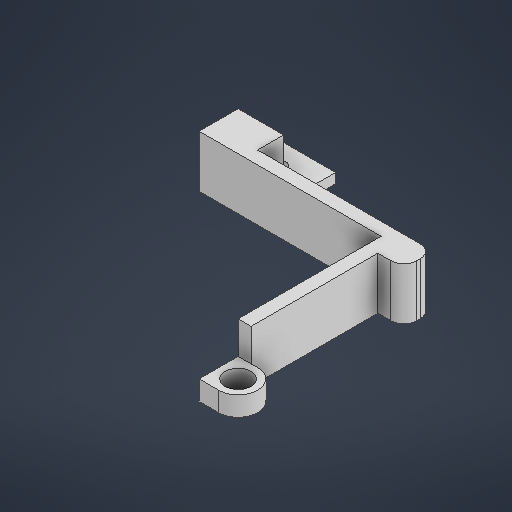
# Autodesk Inventor part: prawascianakolo
Saved by Autodesk Inventor 2026.2 (Build 302298010, 298A)
## iProperties
Created: 2026-04-27
Part Number: prawascianakolo
Material: Ogólny
Document SubType Name: Modeling
Designer: karol
Density: 1 g/cm^3
Appearance: Domyślna
Author: karol
Autodesk Inventor part; units mm, degrees
ref_plane "YZ Plane" through (0, 0, 0) normal (1, 0, 0) x (0, 1, 0)
ref_plane "XZ Plane" through (0, 0, 0) normal (0, 1, 0) x (-1, 0, 0)
ref_plane "XY Plane" through (0, 0, 0) normal (0, 0, 1) x (1, 0, 0)
sketch "Szkic1" plane through (0, 0, 0) normal (0, 1, 0) x (-1, 0, 0)
  line L0 (0, 0) -> (3, 0)
  line L1 (3, 0) -> (3, -25)
  line L2 (3, -25) -> (0, -25)
  line L3 (0, -25) -> (0, 0)
  line L4 (3, -25) -> (31, -25)
  line L5 (31, -25) -> (31, -22)
  line L6 (31, -22) -> (3, -22)
  line L7 (3, -22) -> (3, -25)
  point P0 (3, -22)
  dimension "d0" = 3
  dimension "d1" = 25
  dimension "d2" = 28
  dimension "d3" = 3
  constraints: 16 end point, 4 parallel, 2 horizontal, 2 perpendicular
  measures "d0" distance of L1.end L2.end
  measures "d1" distance of L0.end L1.end
  measures "d2" distance of L6.end L5.end
  measures "d3" distance of L5.end L4.end
extrude "Wyciągnięcie proste1" add sketch "Szkic1" along normal blind 8
sketch "Szkic2" plane through (0, 0, 0) normal (1, 0, 0) x (0, 0, -1)
  line L0 (0, 0) -> (0, 8) projected
  line L1 (0, 8) -> (5, 8)
  line L2 (5, 8) -> (5, 0)
  line L3 (5, 0) -> (0, 0)
  line L4 (0, 0) -> (0, 8)
  dimension "d6" = 5
  dimension "d7" = 8
  constraints: 8 end point, 2 parallel, 1 horizontal, 1 perpendicular
  measures "d6" distance of L2.end L3.end
  measures "d7" distance of L1.end L2.end
extrude "Wyciągnięcie proste2" add sketch "Szkic2" along normal blind 3
sketch "Szkic6" plane through (0, 8, 0) normal (0, 1, 0) x (1, 0, 0)
  line L0 (-31, 22) -> (-3, 22) projected
  line L1 (0, 25) -> (-31, 25) projected
  line L2 (-3, 22) -> (0, 22)
  line L3 (0, 22) -> (0, 25)
  line L4 (0, 25) -> (-3, 25)
  line L5 (-3, 25) -> (-3, 22)
  line L6 (-3, 25) -> (3, 25)
  line L7 (3, 25) -> (3, 19)
  line L8 (3, 19) -> (-3, 19)
  line L9 (-3, 19) -> (-3, 25)
  point P0 (0, 0)
  dimension "d19" = 6
  dimension "d20" = 6
  constraints: 16 end point, 4 parallel, 2 horizontal, 2 perpendicular
  measures "d19" distance of L7.end L8.end
  measures "d20" distance of L6.end L7.end
extrude "Wyciągnięcie proste6" add sketch "Szkic6" against normal blind 8 contours L6 L7 L8 L9 L2 L3
sketch "Szkic7" plane through (0, 8, 0) normal (0, 1, 0) x (1, 0, 0)
  line L0 (3, 19) -> (3, 25) projected
  line L1 (-31, 25) -> (3, 25) projected
  line L2 (-3, 22) -> (-3, 0) projected
  circle A0 centre (0, 22) radius 1.5
  point P0 (0, 0)
  dimension "d23" = 3
  dimension "d42" = 3
  dimension "d43" = 3
  constraints: 1 centre point
  measures "d23" diameter of A0
  measures "d42" distance from line of L1 A0.centre
  measures "d43" distance from line of L2 A0.centre
extrude "Wyciągnięcie proste7" cut sketch "Szkic7" against normal blind 8
sketch "Szkic8" plane through (0, 8, 0) normal (0, 1, 0) x (1, 0, 0)
  circle A0 centre (0, 22) radius 1.5 projected
  circle A1 centre (0, 22) radius 2
  point P0 (0, 0)
  constraints: 1 centre point, 1 coincident
extrude "Wyciągnięcie proste8" add sketch "Szkic8" against normal blind 3 contours A0
sketch "Szkic9" plane through (0, 8, 0) normal (0, 1, 0) x (1, 0, 0)
  line L0 (-31, 25) -> (-31, 22) projected
  line L1 (3, 19) -> (3, 25) projected
  line L2 (-31, 25) -> (3, 25)
  line L3 (3, 25) -> (3, 24)
  line L4 (3, 24) -> (-31, 24)
  line L5 (-31, 24) -> (-31, 25)
  point P0 (0, 0)
  dimension "d28" = 1
  constraints: 8 end point, 2 parallel, 1 horizontal, 1 perpendicular, 1 point on line
  measures "d28" distance of L2.end L3.end
extrude "Wyciągnięcie proste9" cut sketch "Szkic9" against normal blind 8
sketch "Szkic10" plane through (0, 0, -5) normal (0, 0, -1) x (-1, 0, 0)
  line L0 (0, 0) -> (0, 8) projected
  line L1 (-3, 8) -> (-3, 0) projected
  line L2 (0, 0) -> (-3, 0)
  line L3 (-3, 0) -> (-3, 8)
  line L4 (-3, 8) -> (0, 8)
  line L5 (0, 8) -> (0, 0)
  point P0 (-3, 0)
  constraints: 8 end point, 2 parallel, 1 horizontal, 1 perpendicular
extrude "Wyciągnięcie proste10" cut sketch "Szkic10" against normal blind 3.7
sketch "Szkic11" plane through (0, 8, -19) normal (0, 0, 1) x (1, 0, 0)
  line L0 (-3, 0) -> (3, 0) projected
  line L1 (3, -8) -> (0, -8) projected
  line L2 (0, 0) -> (3, 0)
  line L3 (3, 0) -> (3, -8)
  line L4 (3, -8) -> (0, -8)
  line L5 (0, -8) -> (0, 0)
  constraints: 8 end point, 2 parallel, 1 horizontal, 1 midpoint, 1 perpendicular
extrude "Wyciągnięcie proste11" cut sketch "Szkic11" against normal blind 0.5
sketch "Szkic12" plane through (3, 8, -24) normal (0, 0, -1) x (-1, 0, 0)
  line L0 (0, -8) -> (0, 0) projected
  line L1 (6, 0) -> (0, 0) projected
  line L2 (0, -8) -> (6, -8)
  line L3 (6, -8) -> (6, 0)
  line L4 (6, 0) -> (0, 0)
  line L5 (0, 0) -> (0, -8)
  point P0 (3, -8)
  constraints: 8 end point, 2 parallel, 1 horizontal, 1 perpendicular
extrude "Wyciągnięcie proste12" add sketch "Szkic12" along normal blind 0.5
sketch "Szkic13" plane through (0, 0, -1.3) normal (1, 0, 0) x (0, 0, -1)
  line L0 (0, 0) -> (18.2, 0) projected
  line L1 (0, 8) -> (18.2, 8) projected
  line L2 (0, 0) -> (18.2, 0)
  line L3 (18.2, 0) -> (18.2, 8)
  line L4 (18.2, 8) -> (0, 8)
  line L5 (0, 8) -> (0, 0)
  point P0 (-1.3, 0)
  point P1 (18.2, 0)
  constraints: 8 end point, 2 parallel, 1 horizontal, 1 perpendicular
extrude "Wyciągnięcie proste13" cut sketch "Szkic13" against normal blind 1
sketch "Szkic14" plane through (3, 8, -24.5) normal (0, 0, -1) x (-1, 0, 0)
  line L0 (4, 0) -> (0, 0) projected
  line L1 (6, -8) -> (6, 0) projected
  line L2 (0, 0) -> (6, 0)
  line L3 (6, 0) -> (6, -8)
  line L4 (6, -8) -> (0, -8)
  line L5 (0, -8) -> (0, 0)
  point P0 (3, -8)
  constraints: 8 end point, 2 parallel, 1 horizontal, 1 perpendicular
extrude "Wyciągnięcie proste14" cut sketch "Szkic14" against normal blind 0.5
sketch "Szkic15" plane through (-3, 0, 0) normal (0, 0, 1) x (1, 0, 0)
  line L0 (6, 8) -> (6, 0) projected
  line L1 (0, 0) -> (0, 8) projected
  line L2 (6, 8) -> (0, 8)
  line L3 (0, 8) -> (0, 0)
  line L4 (0, 0) -> (6, 0)
  line L5 (6, 0) -> (6, 8)
  point P0 (3, 0)
  constraints: 8 end point, 2 parallel, 1 horizontal, 1 perpendicular
extrude "Wyciągnięcie proste15" add sketch "Szkic15" along normal blind 4.7
sketch "Szkic16" plane through (3, 0, 0) normal (1, 0, 0) x (0, 0, -1)
  line L0 (-4.7, 8) -> (-4.7, 0) projected
  line L1 (1.3, 0) -> (1.3, 8) projected
  line L2 (-4.7, 0) -> (1.3, 0)
  line L3 (1.3, 0) -> (1.3, 8)
  line L4 (1.3, 8) -> (-4.7, 8)
  line L5 (-4.7, 8) -> (-4.7, 0)
  point P0 (0, 0)
  constraints: 8 end point, 2 parallel, 1 horizontal, 1 perpendicular
extrude "Wyciągnięcie proste16" cut sketch "Szkic16" against normal blind 4
sketch "Szkic17" plane through (0, 8, 0) normal (0, 1, 0) x (1, 0, 0)
  line L0 (-1, 19.5) -> (-1, -4.7) projected
  line L1 (-3, -4.7) -> (-1, -4.7)
  line L2 (-1, -4.7) -> (-1, 0)
  line L3 (-1, 0) -> (-3, 0)
  line L4 (-3, 0) -> (-3, -4.7)
  line L5 (-3, 0) -> (3, 0)
  line L6 (3, 0) -> (3, -6)
  line L7 (3, -6) -> (-3, -6)
  line L8 (-3, -6) -> (-3, 0)
  point P0 (0, 0)
  dimension "d48" = 6
  dimension "d49" = 6
  constraints: 16 end point, 4 parallel, 2 horizontal, 2 perpendicular, 1 point on line
  measures "d48" distance of L6.end L7.end
  measures "d49" distance of L5.end L6.end
extrude "Wyciągnięcie proste17" cut sketch "Szkic17" against normal blind 5
sketch "Szkic18" plane through (0, 3, 0) normal (0, 1, 0) x (1, 0, 0)
  line L0 (-3, 0) -> (-1, 0) projected
  line L1 (-3, 0) -> (3, 0)
  line L2 (3, 0) -> (3, -6)
  line L3 (3, -6) -> (-3, -6)
  line L4 (-3, -6) -> (-3, 0)
  point P0 (0, 0)
  dimension "d52" = 6
  dimension "d53" = 6
  constraints: 8 end point, 2 parallel, 1 horizontal, 1 perpendicular
  measures "d52" distance of L2.end L3.end
  measures "d53" distance of L1.end L2.end
extrude "Wyciągnięcie proste18" add sketch "Szkic18" against normal blind 3
sketch "Szkic19" plane through (0, 3, 0) normal (0, 1, 0) x (1, 0, 0)
  circle A0 centre (0, -3) radius 2
  line L0 (-3, -6) -> (-3, 0) projected
  line L1 (-3, -6) -> (3, -6) projected
  point P0 (0, 0)
  dimension "d56" = 4
  dimension "d57" = 3
  dimension "d58" = 3
  constraints: 1 centre point
  measures "d56" diameter of A0
  measures "d57" distance from line of L0 A0.centre
  measures "d58" distance from line of L1 A0.centre
extrude "Wyciągnięcie proste19" cut sketch "Szkic19" against normal blind 3
sketch "Szkic20" plane through (-31, 0, -22) normal (0, 0, 1) x (1, 0, 0)
  line L0 (34, 8) -> (0, 8) projected
  line L1 (0, 8) -> (7, 8)
  line L2 (7, 8) -> (7, 4)
  line L3 (7, 4) -> (0, 4)
  line L4 (0, 4) -> (0, 8)
  point P0 (31, 0)
  point P1 (7, 8)
  dimension "d61" = 7
  dimension "d62" = 4
  constraints: 8 end point, 2 parallel, 1 horizontal, 1 perpendicular
  measures "d61" distance of L2.end L3.end
  measures "d62" distance of L1.end L2.end
extrude "Wyciągnięcie proste20" add sketch "Szkic20" along normal blind 4
sketch "Szkic21" plane through (-31, 0, -24) normal (-1, 0, 0) x (0, 0, 1)
  circle A0 centre (4, 6) radius 1.5
  line L0 (6, 8) -> (6, 4) projected
  line L1 (2, 4) -> (6, 4) projected
  point P0 (24, 0)
  point P1 (4, 4)
  dimension "d65" = 3
  dimension "d66" = 2
  dimension "d67" = 2
  constraints: 1 centre point, 1 midpoint
  measures "d65" diameter of A0
  measures "d66" distance from line of L0 A0.centre
  measures "d67" distance of point (4, 4) A0.centre
extrude "Wyciągnięcie proste21" cut sketch "Szkic21" against normal blind 6
sketch "Szkic22" plane through (3, 8, -24) normal (0, 0, -1) x (-1, 0, 0)
  line L0 (34, 0) -> (34, -8) projected
  line L1 (34, 0) -> (27, 0)
  line L2 (27, 0) -> (27, -4)
  line L3 (27, -4) -> (34, -4)
  line L4 (34, -4) -> (34, 0)
  point P0 (3, -8)
  dimension "d70" = 7
  dimension "d71" = 4
  constraints: 8 end point, 2 parallel, 1 horizontal, 1 perpendicular
  measures "d70" distance of L3.end L2.end
  measures "d71" distance of L2.end L1.end
extrude "Wyciągnięcie proste22" add sketch "Szkic22" along normal blind 4
sketch "Szkic23" plane through (-31, 0, -24) normal (-1, 0, 0) x (0, 0, 1)
  circle A0 centre (-2, 6) radius 1.5
  line L0 (-4, 8) -> (6, 8) projected
  line L1 (-4, 4) -> (-4, 8) projected
  line L2 (2, 0) -> (2, 8) projected
  line L3 (6, 8) -> (2, 8)
  line L4 (2, 8) -> (2, 4)
  line L5 (2, 4) -> (6, 4)
  line L6 (6, 4) -> (6, 8)
  point P0 (24, 0)
  point P1 (-4, 6)
  dimension "d74" = 3
  dimension "d75" = 2
  dimension "d76" = 2
  constraints: 8 end point, 2 midpoint, 2 parallel, 1 centre point, 1 horizontal, 1 perpendicular
  measures "d74" diameter of A0
  measures "d75" distance from line of L0 A0.centre
  measures "d76" distance of point (-4, 6) A0.centre
extrude "Wyciągnięcie proste23" cut sketch "Szkic23" against normal blind 7 contours L0 L6 L5 L2
extrude "Wyciągnięcie proste24" cut sketch "Szkic23" against normal blind 6 contours A0
sketch "Sketch24" plane through (3, 0, -24) normal (0, 0, -1) x (-1, 0, 0)
  line L0 (34, 4) -> (27, 4) projected
  line L1 (27, 4) -> (27, 8) projected
  line L2 (0, 8) -> (27, 8) projected
  line L3 (0, 0) -> (0, 8) projected
  line L4 (34, 0) -> (0, 0) projected
  line L5 (34, 4) -> (34, 0) projected
  point P0 (3, 0)
extrude "Extrusion25" add sketch "Sketch24" along normal blind 0.5
sketch "Szkic25" plane through (3, 0, -24.5) normal (0, 0, -1) x (-1, 0, 0)
  line L0 (27, 4) -> (34, 4) projected
  line L1 (27, 8) -> (27, 4) projected
  line L2 (27, 8) -> (0, 8) projected
  line L3 (0, 8) -> (0, 0) projected
  line L4 (0, 0) -> (34, 0) projected
  line L5 (34, 0) -> (34, 4) projected
  point P0 (3, 0)
extrude "Wyciągnięcie proste26" cut sketch "Szkic25" against normal blind 0.5
sketch "Szkic26" plane through (3, 0, -24) normal (0, 0, -1) x (-1, 0, 0)
  line L0 (34, 0) -> (6, 0) projected
  line L1 (34, 0) -> (24.5, 0)
  line L2 (24.5, 0) -> (24.5, 1.5)
  line L3 (24.5, 1.5) -> (34, 1.5)
  line L4 (34, 1.5) -> (34, 0)
  point P0 (3, 0)
  dimension "d85" = 9.5
  dimension "d86" = 1.5
  constraints: 8 end point, 2 parallel, 1 horizontal, 1 perpendicular
  measures "d85" distance of L2.end L3.end
  measures "d86" distance of L1.end L2.end
extrude "Wyciągnięcie proste27" add sketch "Szkic26" along normal blind 9.5
sketch "Szkic27" plane through (-31, 1.5, -24) normal (0, 1, 0) x (1, 0, 0)
  circle A0 centre (4.26, 6.06) radius 1.05
  line L0 (7, 0) -> (0, 0) projected
  line L1 (0, 0) -> (0, 9.5) projected
  point P0 (31, -24)
  point P1 (0, 4.75)
  dimension "d89" = 2.1
  dimension "d90" = 6.06
  dimension "d91" = 4.26
  constraints: 1 centre point, 1 midpoint
  measures "d89" diameter of A0
  measures "d90" distance from line of L0 A0.centre
  measures "d91" horizontal distance of point (0, 4.75) A0.centre
extrude "Wyciągnięcie proste28" cut sketch "Szkic27" against normal blind 2
fillet "Fillet1" radius 3 2 edges at (3, 1.5, 0) (3, 1.5, 6)
fillet "Fillet2" radius 2 2 edges at (3, 4, -19.5) (3, 4, -24)
